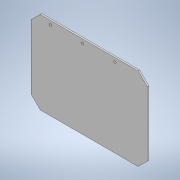
# Autodesk Inventor part: sheetmetalrightside
Saved by Autodesk Inventor 2020.2 (Build 242310000, 310)
## iProperties
Created: 2020-02-05
Part Number: sheetmetalrightside
Material: Generic
Document SubType Name: Sheet Metal
Designer: ColinP
Density: 1 g/cm^3
Sheet Metal Rule: Default
Appearance: Default
Author: ColinP
Autodesk Inventor part; units mm, degrees
ref_plane "YZ Plane" through (0, 0, 0) normal (1, 0, 0) x (0, 1, 0)
ref_plane "XZ Plane" through (0, 0, 0) normal (0, 1, 0) x (-1, 0, 0)
ref_plane "XY Plane" through (0, 0, 0) normal (0, 0, 1) x (1, 0, 0)
sketch "Sketch1" plane through (0, 0, 0) normal (0, 0, 1) x (1, 0, 0)
  line L0 (114.3, 63.5) -> (-114.3, 63.5)
  line L1 (-114.3, 63.5) -> (-114.3, -63.5)
  line L2 (-114.3, -63.5) -> (114.3, -63.5)
  line L3 (114.3, -63.5) -> (114.3, 63.5)
  point P0 (0, 0)
  dimension "d0" = 228.6
  dimension "d1" = 127
  measures "d0" distance of L2.end L1.end
  measures "d1" distance of L1.end L0.end
extrude "Plate1" add sketch "Sketch1" along normal blind 3.048
sketch "Sketch2" plane through (0, 0, 3.048) normal (0, 0, 1) x (1, 0, 0)
  line L0 (114.3, 63.5) -> (-114.3, 63.5)
  line L1 (-114.3, 63.5) -> (-96.3395, 81.4605)
  line L2 (-114.3, 63.5) -> (-88.9, 63.5) construction
  line L3 (114.3, 63.5) -> (96.3395, 81.4605)
  line L4 (114.3, 63.5) -> (139.7, 63.5) construction
  line L5 (96.3395, 81.4605) -> (-96.3395, 81.4605)
  line L6 (-114.3, 63.5) -> (-114.3, -63.5)
  line L7 (-114.3, -63.5) -> (-96.3395, -81.4605)
  line L8 (-114.3, -63.5) -> (-88.9, -63.5) construction
  line L9 (-96.3395, -81.4605) -> (96.3395, -81.4605)
  line L10 (-114.3, -63.5) -> (114.3, -63.5)
  line L11 (96.3395, -81.4605) -> (114.3, -63.5)
  point P0 (0, 0)
  dimension "d3" = 25.4
  dimension "d4" = 45
  dimension "d5" = 25.4
  dimension "d6" = 135
  dimension "d7" = 25.4
  dimension "d8" = 45
  measures "d3" distance of L0.end L1.end
  measures "d4" angle of L2 L1
  measures "d5" distance of L0.start L3.end
  measures "d6" angle of L4 L3
  measures "d7" distance of L6.end L7.end
  measures "d8" angle of L7 L8
sheet face with bend "Face2" sketch "Sketch2" thickness 3.048 toward (0, 0, -1) bend radius 3.048 relief straight relief width 3.048 relief depth 1.524
bend "Bend1"
sketch "Sketch3" plane through (0, 0, 3.048) normal (0, 0, 1) x (1, 0, 0)
  line L0 (-114.3, 63.5) -> (-114.3, -63.5) projected
  line L1 (-114.3, 63.5) -> (-114.3, 57.15)
  line L2 (-114.3, 57.15) -> (114.3, 57.15)
  line L3 (114.3, 63.5) -> (114.3, -63.5) projected
  line L4 (114.3, -63.5) -> (114.3, -57.15)
  line L5 (114.3, -57.15) -> (-114.3, -57.15)
  point P0 (0, 0)
  dimension "d14" = 6.35
  dimension "d15" = 6.35
  constraints: 8 end point, 4 point on line, 2 perpendicular
  measures "d14" distance of L0.start L1.end
  measures "d15" distance of L3.end L4.end
feature "Fold1" [suppressed]
sketch "Sketch4" plane through (0, 0, 3.048) normal (0, 0, 1) x (1, 0, 0)
  line L0 (-114.3, -63.5) -> (-114.3, 63.5) projected
  line L1 (-114.3, -63.5) -> (-114.3, -57.15)
  line L2 (-114.3, -57.15) -> (114.3, -57.15)
  line L3 (114.3, -63.5) -> (114.3, 63.5) projected
  point P0 (0, 0)
  point P1 (-114.3, 53.7028)
  point P2 (114.3, 53.7028)
  dimension "d22" = 6.35
  constraints: 4 end point, 2 point on line, 1 perpendicular
  measures "d22" distance of L0.start L1.end
feature "Fold2" [suppressed]
sketch "Sketch5" plane through (-114.3, 59.7988, 0) normal (0, 1, 0) x (1, 0, 0)
  line L0 (0, 0) -> (0, 107.4056) projected
  line L1 (0, 0) -> (19.05, 0)
  line L2 (0, 0) -> (228.6, 0) projected
  line L3 (19.05, 0) -> (19.05, 25.4)
  line L4 (19.05, 25.4) -> (19.05, 82.4)
  line L5 (19.05, 82.4) -> (64.05, 82.4)
  line L6 (41.55, 82.4) -> (41.55, 77.4)
  line L7 (41.55, 77.4) -> (41.55, 25.4)
  line L8 (41.55, 25.4) -> (41.55, 30.4)
  line L9 (19.05, 25.4) -> (41.55, 25.4)
  line L10 (64.05, 25.4) -> (64.05, 82.4)
  line L11 (64.05, 25.4) -> (41.55, 25.4)
  line L12 (64.05, 82.4) -> (70.4, 82.4)
  line L13 (70.4, 82.4) -> (115.4, 82.4)
  line L14 (115.4, 82.4) -> (115.4, 25.4)
  line L15 (115.4, 25.4) -> (70.4, 25.4)
  line L16 (70.4, 25.4) -> (70.4, 82.4)
  line L17 (92.9, 82.4) -> (92.9, 77.4)
  line L18 (92.9, 77.4) -> (92.9, 30.4)
  dimension "d34" = 19.05
  dimension "d35" = 25.4
  dimension "d36" = 57
  dimension "d37" = 45
  dimension "d38" = 5
  dimension "d39" = 5
  dimension "d40" = 6.35
  dimension "d41" = 45
  dimension "d42" = 5
  dimension "d43" = 47
  constraints: 34 end point, 8 point on line, 6 perpendicular, 3 vertical, 2 horizontal, 2 midpoint
  measures "d34" distance of L0.start L1.end
  measures "d35" distance of L1.end L3.end
  measures "d36" distance of L3.end L4.end
  measures "d37" distance of L4.end L5.end
  measures "d38" distance of L6.start L6.end
  measures "d39" distance of L7.end L8.end
  measures "d40" distance of L5.end L12.end
  measures "d41" distance of L12.end L13.end
  measures "d42" distance of L17.start L17.end
  measures "d43" distance of L17.end L18.end
hole "Hole1" [suppressed]
sketch "Sketch6" plane through (-114.3, 59.7988, 0) normal (0, 1, 0) x (1, 0, 0)
  line L0 (0, 107.4056) -> (228.6, 107.4056) projected
  line L1 (228.6, 107.4056) -> (203.2, 107.4056)
  line L2 (203.2, 107.4056) -> (203.2, 82.0056)
  line L3 (203.2, 82.0056) -> (202.946, 82.0056)
  line L4 (202.946, 82.0056) -> (202.946, 59.0056)
  line L5 (202.946, 59.0056) -> (141.346, 59.0056)
  point P0 (114.3, 0)
  dimension "d51" = 25.4
  dimension "d52" = 25.4
  dimension "d53" = 0.254
  dimension "d54" = 23
  dimension "d55" = 61.6
  constraints: 10 end point, 3 perpendicular, 1 horizontal, 1 point on line
  measures "d51" distance of L0.end L1.end
  measures "d52" distance of L1.end L2.end
  measures "d53" distance of L2.end L3.end
  measures "d54" distance of L3.end L4.end
  measures "d55" distance of L4.end L5.end
hole "Hole2" [suppressed]
sketch "Sketch7" plane through (96.3395, 81.4605, 0) normal (0, 0, 1) x (-1, 0, 0)
  line L0 (-17.9605, 17.9605) -> (0, 0) projected
  line L1 (-17.9605, 17.9605) -> (-17.9605, 7.8005)
  line L2 (-17.9605, 17.9605) -> (-7.8005, 17.9605) construction
  line L3 (-17.9605, 7.8005) -> (45.5395, 7.8005)
  line L4 (45.5395, 7.8005) -> (109.0395, 7.8005)
  line L5 (109.0395, 7.8005) -> (172.5395, 7.8005)
  line L6 (172.5395, 7.8005) -> (236.0395, 7.8005)
  point P0 (96.3395, 81.4605)
  dimension "d63" = 10.16
  dimension "d64" = 90
  dimension "d65" = 63.5
  dimension "d66" = 63.5
  dimension "d67" = 63.5
  dimension "d68" = 180
  dimension "d69" = 63.5
  constraints: 12 end point, 2 horizontal, 2 point on line, 1 collinear, 1 perpendicular, 1 vertical
  measures "d63" distance of L0.start L1.end
  measures "d64" angle of L1 L2
  measures "d65" distance of L1.end L3.end
  measures "d66" distance of L3.end L4.end
  measures "d67" distance of L4.end L5.end
  measures "d68" angle of L5 L4
  measures "d69" distance of L5.end L6.end
hole "Hole3" at (50.8, 73.66, 0) at (-12.7, 73.66, 0) at (-76.2, 73.66, 0) direction (0, 0, 1) diameter 4.4958 end through all clearance for "Flat Head Machine Screw (82)" size "#8" standard "Ansi Unified Screw Threads"
sketch "Sketch8" plane through (114.3, -57.5492, 6.096) normal (0, -1, 0) x (1, 0, 0)
  line L0 (-113.2, 25.0056) -> (-113.2, 82.0056) projected
  line L1 (-158.2, 25.0056) -> (-113.2, 25.0056) projected
  line L2 (-113.2, 82.0056) -> (-158.2, 82.0056) projected
  line L3 (-158.2, 82.0056) -> (-158.2, 25.0056) projected
  line L4 (-164.55, 25.0056) -> (-158.2, 25.0056) projected
  line L5 (-135.7, 30.0056) -> (-135.7, 77.0056) projected
  line L6 (-17.9605, -6.096) -> (0, -6.096) projected
  line L7 (-210.6395, -6.096) -> (-17.9605, -6.096) projected
  line L8 (-228.6, -6.096) -> (-210.6395, -6.096) projected
  line L9 (-210.6395, -6.096) -> (-228.6, -6.096) projected
  line L10 (-17.9605, -6.096) -> (-210.6395, -6.096) projected
  line L11 (0, -6.096) -> (-17.9605, -6.096) projected
  point P0 (-114.3, -6.096)
equation "\"d2\" = Thickness"
equation "\"d16\" = BendReliefWidth"
equation "\"d17\" = BendReliefDepth"
equation "\"d18\" = MinimumRemnant"
equation "\"d19\" = TransitionRadius"
equation "\"d21\" = BendRadius"
equation "\"d23\" = BendReliefWidth"
equation "\"d24\" = BendReliefDepth"
equation "\"d25\" = MinimumRemnant"
equation "\"d26\" = TransitionRadius"
equation "\"d28\" = BendRadius"
equation "\"d49\" = Thickness"
equation "\"d61\" = Thickness"
equation "\"d75\" = Thickness"
equation "\"d9\" = BendRadius"
equation "\"d10\" = BendReliefWidth"
equation "\"d12\" = MinimumRemnant"
equation "\"d11\" = BendReliefDepth"
equation "\"d13\" = TransitionRadius"
equation "\"BendRadius\" = Thickness"
equation "\"BendReliefWidth\" = Thickness"
equation "\"BendReliefDepth\" = 0.5 * Thickness"
equation "\"CornerReliefSize\" = 4 * Thickness"
equation "\"MinimumRemnant\" = 2 * Thickness"
equation "\"TransitionRadius\" = BendRadius"
equation "\"JacobiRadiusSize\" = BendRadius"
equation "\"GapSize\" = Thickness"
equation "\"Thickness\" = 3.048"
body "Solid1"
